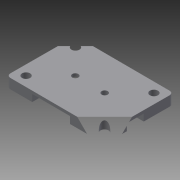
# Autodesk Inventor part: GehäuseBack
Saved by Autodesk Inventor 2014 (Build 180170000, 170)
## iProperties
Created: 2013-05-31
Part Number: GehäuseBack
Material: Generisch
Document SubType Name: Modeling
Designer: hanse
Density: 1 g/cm^3
Appearance: Vorgabe
Author: hanse
Autodesk Inventor part; units mm, degrees
ref_plane "YZ Plane" through (0, 0, 0) normal (1, 0, 0) x (0, 1, 0)
ref_plane "XZ Plane" through (0, 0, 0) normal (0, 1, 0) x (-1, 0, 0)
ref_plane "XY Plane" through (0, 0, 0) normal (0, 0, 1) x (1, 0, 0)
sketch "Skizze1" plane through (0, 0, 0) normal (0, 0, 1) x (1, 0, 0)
  line L0 (17.6969, -0.7673) -> (8.7277, -0.7347) projected
  arc A0 (8.2588, 6.1863) -> (8.7277, -0.7347) centre (0.2074, 2.1644) ccw projected
  line L1 (8.2588, 6.1863) -> (17.722, 6.1519) projected
  line L2 (17.7709, 19.6007) -> (17.722, 6.1519) projected
  line L3 (-32.2287, 19.7825) -> (17.7709, 19.6007) projected
  line L4 (-32.356, -15.2173) -> (-32.2287, 19.7825) projected
  line L5 (17.6436, -15.3991) -> (-32.356, -15.2173) projected
  line L6 (17.6969, -0.7673) -> (17.6436, -15.3991) projected
  circle A1 centre (-14.7925, 2.219) radius 1.45 projected
  circle A2 centre (-14.7925, 2.219) radius 1.55
  circle A3 centre (0.2074, 2.1644) radius 1.55
  line L7 (17.6969, -0.7673) -> (17.722, 6.1519)
  circle A4 centre (-27.247, 14.7644) radius 2.05 projected
  circle A5 centre (12.6619, -10.381) radius 2.05 projected
  circle A6 centre (12.7528, 14.6189) radius 2.05 projected
  circle A7 centre (-27.3379, -10.2355) radius 2.05 projected
  point P0 (0, 0)
  dimension "d25" = 3.1
  dimension "d26" = 3.1
  constraints: 2 centre point, 2 coincident, 2 end point, 1 collinear
  measures "d25" diameter of A2
  measures "d26" diameter of A3
extrude "Extrusion1" add sketch "Skizze1" along normal blind 1.5 contours L6 L5 L4 L3 L2 L1 A0 L0 | L0 A0 L1 L7
sketch "Skizze6" plane through (0, 0, 0) normal (0, 0, -1) x (-1, 0, 0)
  circle A0 centre (14.7925, 2.219) radius 1.55 projected
  circle A1 centre (-0.2074, 2.1644) radius 1.55 projected
  circle A2 centre (-0.2074, 2.1644) radius 14.0891
  circle A3 centre (14.7925, 2.219) radius 14.0891
  line L0 (32.356, -15.2173) -> (-17.6436, -15.3991) projected
  line L1 (32.2287, 19.7825) -> (32.356, -15.2173) projected
  line L2 (-17.7709, 19.6007) -> (32.2287, 19.7825) projected
  line L3 (-17.6436, -15.3991) -> (-17.7709, 19.6007)
  line L4 (32.2287, 19.7825) -> (-17.7709, 19.6007)
  line L5 (32.356, -15.2173) -> (32.2287, 19.7825)
  line L6 (32.356, -15.2173) -> (-17.6436, -15.3991)
  circle A4 centre (27.3379, -10.2355) radius 2.05 projected
  circle A5 centre (-12.7528, 14.6189) radius 2.05 projected
  circle A6 centre (-12.6619, -10.381) radius 2.05 projected
  circle A7 centre (27.247, 14.7644) radius 2.05 projected
  circle A8 centre (-12.7528, 14.6189) radius 2.05
  circle A9 centre (27.247, 14.7644) radius 2.05
  circle A10 centre (27.3379, -10.2355) radius 2.05
  circle A11 centre (-12.6619, -10.381) radius 2.05
  point P0 (0, 0)
  constraints: 8 end point, 6 centre point, 6 coincident, 5 equal radius, 3 collinear, 1 perpendicular
extrude "Extrusion7" add sketch "Skizze6" along normal blind 3.5
sketch "Skizze7" plane through (0, 0, -3.5) normal (0, 0, -1) x (-1, 0, 0)
  line L0 (-21.514, 4.474) -> (38.6582, 4.474)
  line L1 (38.6582, 4.474) -> (38.6582, -4.0646)
  line L2 (38.6582, -4.0646) -> (-21.514, -4.0646)
  line L3 (-21.514, -4.0646) -> (-21.514, 4.474)
  line L4 (-0.0651, 23.7233) -> (19.1842, 23.7233)
  line L5 (19.1842, 23.7233) -> (19.1842, -21.5163)
  line L6 (19.1842, -21.5163) -> (-0.0651, -21.5163)
  line L7 (-0.0651, -21.5163) -> (-0.0651, 23.7233)
  point P0 (0, 0)
  constraints: 16 end point, 4 parallel, 2 horizontal, 2 perpendicular
extrude "Extrusion8" cut sketch "Skizze7" against normal up to surface (3.5 mm away)
sketch "Skizze2" plane through (0, 0, 0) normal (0, 0, -1) x (-1, 0, 0)
  circle A0 centre (-0.2074, 2.1644) radius 1.55 projected
  arc A1 (-12.8448, -4.0646) -> (-0.0651, -11.924) centre (-0.2074, 2.1644) ccw projected
  circle A2 centre (-0.2074, 2.1644) radius 3.55
  point P0 (0, 0)
  dimension "d27" = 2
  constraints: 1 centre point, 1 coincident
  measures "d27" radial gap between concentric circles of A2 A0
extrude "Extrusion2" add sketch "Skizze2" along normal blind 3.5
fillet "Rundung5" radius 2 4 edges at (3.7574, 2.1644, 0) (-32.356, -15.2173, -1) (17.7709, 19.6007, -1) (-32.2287, 19.7825, -1)
